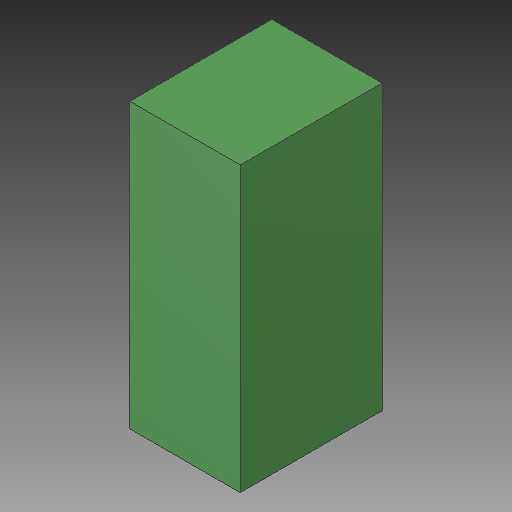
# Autodesk Inventor part: PZT
Saved by Autodesk Inventor 2019.2 (Build 232265000, 265)
## iProperties
Created: 2018-03-05
Part Number: PZT
Material: Generic
Document SubType Name: Modeling
Designer: Hogar
Density: 1 g/cm^3
Appearance: Default
Author: Hogar
Autodesk Inventor part; units mm, degrees
ref_plane "YZ Plane" through (0, 0, 0) normal (1, 0, 0) x (0, 1, 0)
ref_plane "XZ Plane" through (0, 0, 0) normal (0, 1, 0) x (-1, 0, 0)
ref_plane "XY Plane" through (0, 0, 0) normal (0, 0, 1) x (1, 0, 0)
sketch "Sketch1" plane through (0, 0, 0) normal (0, 0, 1) x (1, 0, 0)
  line L0 (-1.75, -4.5) -> (1.75, -4.5)
  line L1 (1.75, -4.5) -> (1.75, 4.5)
  line L2 (1.75, 4.5) -> (-1.75, 4.5)
  line L3 (-1.75, 4.5) -> (-1.75, -4.5)
  line L4 (-1.75, -4.5) -> (1.75, 4.5) construction
  line L5 (1.75, -4.5) -> (-1.75, 4.5) construction
  point P0 (0, 0)
  dimension "d0" = 3.5
  dimension "d1" = 9
  constraints: 12 end point, 2 midpoint, 2 parallel, 1 horizontal, 1 perpendicular
  measures "d0" distance of L2.end L1.end
  measures "d1" distance of L1.end L0.end
extrude "Extrusion1" add sketch "Sketch1" along normal blind 4.5
ref_plane "Work Plane1" through (-1.75, -4.5, 0) normal (0, -1, 0) x (1, 0, 0)
ref_plane "Work Plane2" through (0, 0, 2.25) normal (0, 0, 1) x (1, 0, 0)
body "Solid1"
